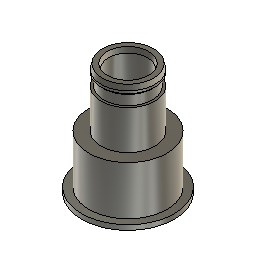
Schlauchadapter-22mm-40mm NATO (Autodesk Fusion 360 design; units mm, degrees)
Autodesk Fusion 360 part; units mm, degrees
sketch "Skizze1" plane through (0, 0, 0) normal (1, 0, 0) x (0, 1, 0) in component "Schlauchadapter-22mm-40mm NATO"
  line L0 (0, -8) -> (0, 92) construction
  line L1 (0, 0) -> (19, 0) construction
  line L2 (13.5, -8.8503) -> (13.5, 10.0011) construction
  line L3 (16, -9) -> (16, -8)
  line L4 (16, -8) -> (16, 12.6517) construction
  line L5 (8, 9.6655) -> (8, 11)
  line L6 (8, 11) -> (8, 32.4994) construction
  line L7 (13.5, 0) -> (19, 0)
  line L8 (19, 0) -> (19, 2)
  line L9 (19, 2) -> (16, 2)
  line L10 (16, 2) -> (16, 22)
  line L11 (13.5, 0) -> (13.5, 5)
  line L12 (16, 22) -> (-10.2408, 22) construction
  line L13 (11, 9.9222) -> (11, 30.0778) construction
  line L14 (16, 22) -> (11, 22)
  line L15 (11, 22) -> (11, 38)
  line L16 (8, 28.4613) -> (8, 38.3723) construction
  line L17 (10, 31.378) -> (10, 40.0422) construction
  line L18 (11, 38) -> (10, 38)
  line L19 (10, 38) -> (10, 42)
  line L20 (11, 38) -> (-2.5, 38) construction
  line L21 (8, 22) -> (8, 38)
  line L22 (11, 22) -> (11, 43) construction
  line L23 (10, 42) -> (11, 42)
  line L24 (11, 42) -> (11, 46)
  line L25 (11, 46) -> (8, 46)
  line L26 (8, 46) -> (8, 38)
  line L27 (8, 22) -> (13.5, 5)
  dimension "d16" = 19
  dimension "d17" = 13.5
  dimension "d18" = 16
  dimension "d19" = 8
  dimension "d20" = 2
  dimension "d21" = 20
  dimension "d22" = 5
  dimension "d23" = 11
  dimension "d24" = 16
  dimension "d25" = 8
  dimension "d26" = 10
  dimension "d27" = 4
  dimension "d28" = 4
  constraint vertical L0
  constraint coincident L1.start origin
  constraint perpendicular L0 L1
  constraint parallel L0 L2
  constraint vertical L3
  constraint parallel L0 L4
  constraint vertical L5
  constraint parallel L0 L6
  constraint coincident L1 L7.start
  constraint coincident L2 L7.start
  constraint perpendicular L1 L8
  constraint coincident L4 L9.end
  constraint perpendicular L4 L9
  constraint perpendicular L9 L10
  constraint perpendicular L1 L11
  constraint perpendicular L10 L12
  constraint coincident L6 L21.start
  constraint coincident L12 L21.start
  constraint parallel L0 L13
  constraint coincident L12 L14.end
  constraint coincident L13 L14.end
  constraint perpendicular L12 L15
  constraint parallel L0 L16
  constraint parallel L0 L17
  constraint coincident L17 L18.end
  constraint perpendicular L17 L18
  constraint perpendicular L18 L19
  constraint perpendicular L0 L20
  constraint coincident L20 L21.end
  constraint coincident L16 L21.end
  constraint perpendicular L14 L22
  constraint coincident L22 L23.end
  constraint perpendicular L22 L23
  constraint perpendicular L23 L24
  constraint perpendicular L24 L25
  constraint perpendicular L20 L26
  measures "d16" distance of L1.start L1.end
  measures "d17" distance of L0 L2
  measures "d18" distance of L0 L4
  measures "d19" distance of L0 L6
  measures "d20" distance of L1.end L8.end
  measures "d21" distance of L9.end L10.end
  measures "d22" distance of L7.start L11.end
  measures "d23" distance of L0 L13
  measures "d24" distance of L14.end L15.end
  measures "d25" distance of L0 L16
  measures "d26" distance of L0 L17
  measures "d27" distance of L18.end L19.end
  measures "d28" distance of L23.end L24.end
revolve "Drehen1" add sketch "Skizze1" angle 360 about axis through (0, 0, -8) along (0, 0, 1) in component "Schlauchadapter-22mm-40mm NATO"
chamfer "Fase1" distance 2 distance2 0.5 1 edges at (-10.2556, 3.9778, 46) measured on face at (0.5483, 10.9863, 43.3333) in component "Schlauchadapter-22mm-40mm NATO"
chamfer "Fase2" distance 1 angle 45 1 edges at (-10.2556, 3.9778, 42) in component "Schlauchadapter-22mm-40mm NATO"
chamfer "Fase4" distance 0.5 distance2 2 1 edges at (-7.4586, 2.8929, 46) measured on face at (0.9191, 9.5978, 46) in component "Schlauchadapter-22mm-40mm NATO"
component "Schlauchadapter-22mm-40mm NATO" placed x (1, 0, 0) y (0, 1, 0) z (0, 0, 1) at (0, 0, 0)
